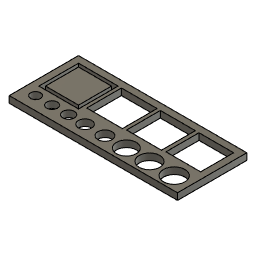
ToleranceTool (Autodesk Fusion 360 design; units mm, degrees)
Autodesk Fusion 360 part; units mm, degrees
sketch "Sketch1" plane through (0, 0, 0) normal (0, 1, 0) x (1, 0, 0)
  line L0 (51, 21) -> (0, 21)
  line L1 (0, 21) -> (0, 0)
  circle A0 centre (4, 4) radius 1.5
  circle A1 centre (9, 4) radius 1.625
  circle A2 centre (14, 4) radius 1.75
  circle A3 centre (19, 4) radius 2
  circle A4 centre (25, 4) radius 2.125
  line L2 (38.5, 19) -> (49, 19)
  line L3 (49, 19) -> (49, 9)
  line L4 (49, 9) -> (38.5, 9)
  line L5 (38.5, 9) -> (38.5, 19)
  line L6 (26.8, 19) -> (37.4, 19)
  line L7 (37.4, 19) -> (37.4, 8.75)
  line L8 (37.4, 8.75) -> (26.8, 8.75)
  line L9 (26.8, 8.75) -> (26.8, 19)
  line L10 (15, 19) -> (25.8, 19)
  line L11 (25.8, 19) -> (25.8, 8.5)
  line L12 (25.8, 8.5) -> (15, 8.5)
  line L13 (15, 8.5) -> (15, 19)
  line L14 (3, 18) -> (13, 18)
  line L15 (13, 18) -> (13, 8)
  line L16 (13, 8) -> (3, 8)
  line L17 (3, 8) -> (3, 18)
  line L18 (2, 7) -> (14, 7)
  line L19 (14, 7) -> (14, 19)
  line L20 (14, 19) -> (2, 19)
  line L21 (2, 19) -> (2, 7)
  circle A5 centre (31.5, 4) radius 3
  line L22 (0, 0) -> (51, 0)
  line L23 (51, 0) -> (51, 8)
  line L24 (51, 8) -> (51, 21)
  line L25 (2, 19) -> (14, 7) construction
  line L26 (13, 18) -> (3, 8) construction
  line L27 (0, 4) -> (51, 4) construction
  circle A6 centre (38.5, 4) radius 3.125
  circle A7 centre (46, 4) radius 3.25
  point P0 (8, 13)
  point P1 (8, 13)
  dimension "d1" = 3
  dimension "d2" = 3.25
  dimension "d3" = 3.5
  dimension "d4" = 4
  dimension "d5" = 4.25
  dimension "d6" = 10.25
  dimension "d7" = 10.5
  dimension "d8" = 10
  dimension "d9" = 10
  dimension "d10" = 12
  dimension "d11" = 12
  dimension "d12" = 6
  dimension "d13" = 10.8
  dimension "d14" = 10.6
  dimension "d15" = 10.5
  dimension "d16" = 10
  dimension "d17" = 2
  dimension "d18" = 2
  dimension "d19" = 2
  dimension "d20" = 13
  dimension "d21" = 51
  dimension "d22" = 21
  dimension "d23" = 1
  dimension "d24" = 1
  dimension "d25" = 1.1
  dimension "d26" = 4
  dimension "d27" = 9
  dimension "d28" = 14
  dimension "d29" = 19
  dimension "d30" = 25
  dimension "d31" = 31.5
  dimension "d32" = 6.25
  dimension "d33" = 6.5
  dimension "d34" = 38.5
  dimension "d35" = 46
  constraint vertical L1
  constraint coincident L1.end L22.start
  constraint horizontal L2
  constraint vertical L3
  constraint horizontal L4
  constraint vertical L5
  constraint horizontal L6
  constraint vertical L7
  constraint horizontal L8
  constraint vertical L9
  constraint horizontal L10
  constraint vertical L11
  constraint horizontal L12
  constraint vertical L13
  constraint horizontal L14
  constraint vertical L15
  constraint horizontal L16
  constraint vertical L17
  constraint horizontal L18
  constraint vertical L19
  constraint horizontal L20
  constraint vertical L21
  constraint perpendicular L1 L22
  constraint vertical L0.start L23.end
  constraint collinear L10 L20
  constraint collinear L6 L20
  constraint collinear L2 L20
  constraint midpoint L26 P1
  constraint midpoint L25 P1
  constraint coincident P1 P0
  constraint coincident L1 L27.start
  constraint coincident L23 L27.end
  constraint perpendicular L1 L27
  constraint midpoint L23 L27.end
  constraint coincident A5.centre L27
  constraint coincident A4.centre L27
  constraint coincident A3.centre L27
  constraint coincident A2.centre L27
  constraint coincident A1.centre L27
  constraint coincident A0.centre L27
  constraint coincident L27 A6.centre
  constraint coincident L27 A7.centre
  constraint parallel L23 L24
  measures "d1" diameter of A0
  measures "d2" diameter of A1
  measures "d3" diameter of A2
  measures "d4" diameter of A3
  measures "d5" diameter of A4
  measures "d6" distance of L6.start L8.end
  measures "d7" distance of L10.start L12.end
  measures "d8" distance of L14.start L16.end
  measures "d9" distance of L14.start L14.end
  measures "d10" distance of L19.end L20.end
  measures "d11" distance of L18.end L19.end
  measures "d12" diameter of A5
  measures "d13" distance of L11.end L12.end
  measures "d14" distance of L7.end L8.end
  measures "d15" distance of L3.end L4.end
  measures "d16" distance of L2.end L3.end
  measures "d17" distance of L1 L21
  measures "d18" distance of L0 L20
  measures "d19" distance of L3 L24
  measures "d20" distance of L0.start L23.end
  measures "d21" distance of L0.start L0.end
  measures "d22" distance of L1.end L0.end
  measures "d23" distance of L13 L19
  measures "d24" distance of L9 L11
  measures "d25" distance of L5 L7
  measures "d26" distance of L1 A0.centre
  measures "d27" distance of L1 A1.centre
  measures "d28" distance of L1 A2.centre
  measures "d29" distance of L1 A3.centre
  measures "d30" distance of L1 A4.centre
  measures "d31" distance of L1 A5.centre
  measures "d32" diameter of A6
  measures "d33" diameter of A7
  measures "d34" distance of L1 A6.centre
  measures "d35" distance of L1 A7.centre
extrude "Extrude1" add sketch "Sketch1" along normal blind 2 makes body 1 at (20.0817, 0, -7.65) makes body 2 at (6.3333, 0, -14.6667)
